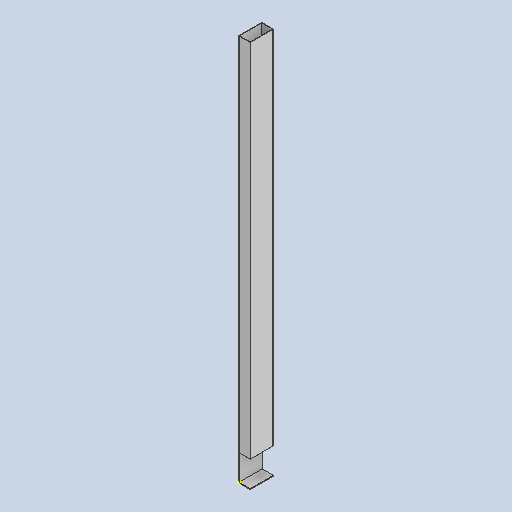
# Autodesk Inventor part: Expendedor
Saved by Autodesk Inventor 2026 (Build 300175050, 175E)
## iProperties
Created: 2025-10-30
Part Number: Expendedor
Material: Genérico
Document SubType Name: Modeling
Designer: bello
Density: 1 g/cm^3
Appearance: Valor por defecto
Author: bello
Autodesk Inventor part; units mm, degrees
ref_plane "YZ Plane" through (0, 0, 0) normal (1, 0, 0) x (0, 1, 0)
ref_plane "XZ Plane" through (0, 0, 0) normal (0, 1, 0) x (-1, 0, 0)
ref_plane "XY Plane" through (0, 0, 0) normal (0, 0, 1) x (1, 0, 0)
sketch "Boceto1" plane through (0, 0, 0) normal (0, 1, 0) x (-1, 0, 0)
  line L0 (0, 0) -> (30, 0)
  line L1 (30, 0) -> (30, -60)
  line L2 (30, -60) -> (0, -60)
  line L3 (0, -60) -> (0, 0)
  dimension "d0" = 60
  dimension "d1" = 30
  constraints: 8 end point, 2 parallel, 1 horizontal, 1 perpendicular
  measures "d0" distance of L0.end L1.end
  measures "d1" distance of L1.end L2.end
extrude "Extrusión1" add sketch "Boceto1" along normal blind 1000
sketch "Boceto2" plane through (0, 0, 0) normal (0, -1, 0) x (1, 0, 0)
  line L0 (-1.2, -1.2) -> (-28.8, -1.2)
  line L1 (-28.8, -1.2) -> (-28.8, -58.8)
  line L2 (-28.8, -58.8) -> (-1.2, -58.8)
  line L3 (-1.2, -58.8) -> (-1.2, -1.2)
  line L4 (0, 0) -> (0, -60) projected
  line L5 (-30, -60) -> (-30, 0) projected
  line L6 (-30, 0) -> (0, 0) projected
  line L7 (0, -60) -> (-30, -60) projected
  dimension "d4" = 1.2
  dimension "d5" = 1.2
  dimension "d6" = 1.2
  dimension "d7" = 1.2
  constraints: 8 end point, 2 parallel, 1 horizontal, 1 perpendicular
  measures "d4" distance between parallel lines of L3 L4
  measures "d5" distance between parallel lines of L5 L1
  measures "d6" distance between parallel lines of L6 L0
  measures "d7" distance between parallel lines of L7 L2
extrude "Extrusión2" cut sketch "Boceto2" against normal through all contours L3 L2 L1 L0
sketch "Boceto3" plane through (-30, 0, 0) normal (0, 0, 1) x (1, 0, 0)
  line L0 (30, 0) -> (1.2, 0)
  line L1 (1.2, 0) -> (1.2, 66)
  line L2 (1.2, 66) -> (30, 66)
  line L3 (30, 66) -> (30, 0)
  line L4 (0, 0) -> (0, 1000) projected
  dimension "d10" = 1.2
  dimension "d11" = 66
  constraints: 8 end point, 2 parallel, 1 horizontal, 1 perpendicular
  measures "d10" distance between parallel lines of L4 L1
  measures "d11" distance of L2.end L0.start
extrude "Extrusión3" cut sketch "Boceto3" against normal through all
sketch "Boceto4" plane through (-28.8, 0, 0) normal (1, 0, 0) x (0, 0, -1)
  point P0 (0, 0)
sketch "Boceto5" plane through (-30, 0, -60) normal (-1, 0, 0) x (0, 0, 1)
  line L0 (60, 0) -> (0, 0)
  line L1 (0, 0) -> (0, -2)
  line L2 (0, -2) -> (60, -2)
  line L3 (60, -2) -> (60, 0)
  dimension "d14" = 2
  constraints: 8 end point, 2 parallel, 1 horizontal, 1 perpendicular
  measures "d14" distance of L2.end L0.start
extrude "Extrusión4" add sketch "Boceto5" against normal blind 30
